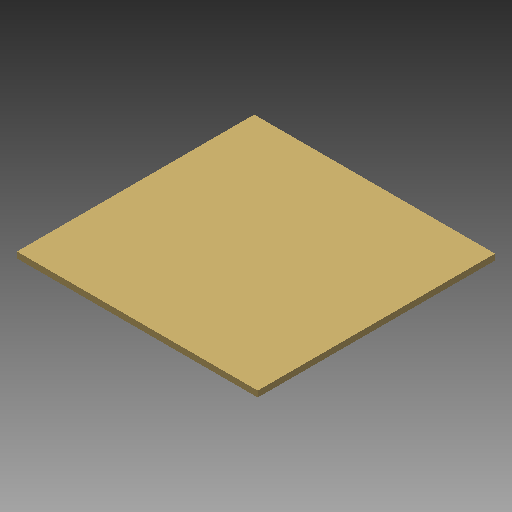
# Autodesk Inventor part: Pianka_oparcia
Saved by Autodesk Inventor 2017 (Build 210142000, 142)
## iProperties
Created: 2015-12-07
Part Number: Pianka_oparcia
Material: Pianka poliuretanowa
Document SubType Name: Modeling
Designer: graaapsik
Density: 0.02 g/cm^3
Appearance: Pianka poliuretanowa
Mass: 32.319 g
Surface Area: 3392.7 cm^2
Volume: 1615.95 cm^3
Author: graaapsik
Autodesk Inventor part; units mm, degrees
ref_plane "YZ Plane" through (0, 0, 0) normal (1, 0, 0) x (0, 1, 0)
ref_plane "XZ Plane" through (0, 0, 0) normal (0, 1, 0) x (-1, 0, 0)
ref_plane "XY Plane" through (0, 0, 0) normal (0, 0, 1) x (1, 0, 0)
sketch "Szkic1" plane through (0, 0, 0) normal (0, 0, 1) x (1, 0, 0)
  line L0 (0, 0) -> (405, 0)
  line L1 (405, 0) -> (405, 10)
  line L2 (405, 10) -> (0, 10)
  line L3 (0, 10) -> (0, 0)
  dimension "d0" = 405
  dimension "d1" = 10
  constraints: 8 end point, 2 parallel, 1 horizontal, 1 perpendicular
  measures "d0" distance of L0.start L0.end
  measures "d1" distance of L2.end L0.start
extrude "Wyciągnięcie proste1" add sketch "Szkic1" along normal mid plane 399
